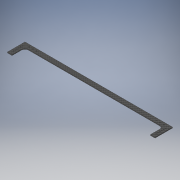
# Autodesk Inventor part: Brace 1
Saved by Autodesk Inventor 2019.4 (Build 234330000, 330)
## iProperties
Created: 2019-12-14
Part Number: Brace 1
Material: CFRP
Document SubType Name: Modeling
Designer: admin
Density: 1.43 g/cm^3
Appearance: Carbon Fiber
Author: admin
Autodesk Inventor part; units mm, degrees
ref_plane "YZ Plane" through (0, 0, 0) normal (1, 0, 0) x (0, 1, 0)
ref_plane "XZ Plane" through (0, 0, 0) normal (0, 1, 0) x (-1, 0, 0)
ref_plane "XY Plane" through (0, 0, 0) normal (0, 0, 1) x (1, 0, 0)
sketch "Sketch1" plane through (0, 0, 0) normal (0, 1, 0) x (-1, 0, 0)
  line L0 (0, 0) -> (0, -95)
  line L1 (0, -95) -> (-95, -95)
  line L2 (-95, -95) -> (-95, -70) construction
  line L3 (-95, -70) -> (-25, -70)
  line L4 (-25, -70) -> (-25, 0)
  line L5 (-25, 0) -> (0, 0)
  circle A0 centre (-12.5, -20) radius 2.75
  line L6 (-12.5, 0) -> (-12.5, -95) construction
  circle A1 centre (-12.5, -40) radius 2.75
  circle A2 centre (-12.5, -60) radius 2.75
  line L7 (-95, -82.5) -> (0, -82.5) construction
  circle A3 centre (-35, -82.5) radius 2.75
  circle A4 centre (-55, -82.5) radius 2.75
  circle A5 centre (-75, -82.5) radius 2.75
  circle A6 centre (-12.5, -30) radius 2.75
  circle A7 centre (-12.5, -50) radius 2.75
  circle A8 centre (-12.5, -70) radius 2.75
  line L8 (-400, -139.4226) -> (-400, 36.9661) construction
  line L9 (-800, 0) -> (-800, -95)
  line L10 (-800, -95) -> (-705, -95)
  line L11 (-705, -95) -> (-705, -70) construction
  line L12 (-705, -70) -> (-775, -70)
  line L13 (-775, -70) -> (-775, 0)
  line L14 (-775, 0) -> (-800, 0)
  circle A9 centre (-787.5, -20) radius 2.75
  line L15 (-787.5, 0) -> (-787.5, -95) construction
  circle A10 centre (-787.5, -40) radius 2.75
  circle A11 centre (-787.5, -60) radius 2.75
  line L16 (-705, -82.5) -> (-800, -82.5) construction
  circle A12 centre (-765, -82.5) radius 2.75
  circle A13 centre (-745, -82.5) radius 2.75
  circle A14 centre (-725, -82.5) radius 2.75
  circle A15 centre (-787.5, -30) radius 2.75
  circle A16 centre (-787.5, -50) radius 2.75
  circle A17 centre (-787.5, -70) radius 2.75
  line L17 (-95, -95) -> (-705, -95)
  line L18 (-705, -70) -> (-95, -70)
  dimension "d0" = 25
  dimension "d1" = 70
  dimension "d2" = 25
  dimension "d3" = 70
  dimension "d4" = 5.5
  dimension "d5" = 20
  dimension "d6" = 5.5
  dimension "d7" = 5.5
  dimension "d8" = 20
  dimension "d9" = 20
  dimension "d12" = 5.5
  dimension "d13" = 35
  dimension "d14" = 5.5
  dimension "d15" = 20
  dimension "d16" = 5.5
  dimension "d17" = 20
  dimension "d22" = 10
  dimension "d28" = 400
  constraints: 38 end point, 19 symmetric about line, 18 centre point, 16 point on line, 7 perpendicular, 3 vertical, 2 midpoint, 1 horizontal, 1 parallel, 15 other
  measures "d0" distance between parallel lines of L0 L4
  measures "d1" distance of L3.end L4.end
  measures "d2" distance of L1.end L2.end
  measures "d3" distance of L2.end L3.end
  measures "d4" diameter of A0
  measures "d5" distance from line of L5 A0.centre
  measures "d6" diameter of A1
  measures "d7" diameter of A2
  measures "d8" distance of A0.centre A1.centre
  measures "d9" distance of A1.centre A2.centre
  measures "d12" diameter of A3
  measures "d13" distance from line of L0 A3.centre
  measures "d14" diameter of A4
  measures "d15" distance of A3.centre A4.centre
  measures "d16" diameter of A5
  measures "d17" distance of A4.centre A5.centre
  measures "d22" distance of A0.centre A6.centre
  measures "d28" distance between parallel lines of L8 L0
extrude "Extrusion1" add sketch "Sketch1" along normal blind 4
fillet "Fillet1" radius 20 2 edges at (25, 2, -70) (775, 2, -70)
body "Solid1"
